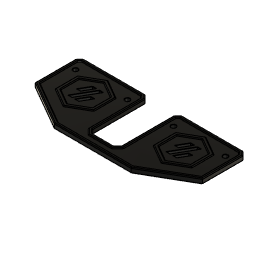
z_chain_cover (Autodesk Fusion 360 design; units mm, degrees)
Autodesk Fusion 360 part; units mm, degrees
note: some values were not read from the file. Chosen so that the rebuilt part matches the saved one: which pieces of a blend or face edit are solid. Set by a fixed rule: which sketch regions a step uses.
sketch "Sketch1" plane through (0, 0, 0) normal (0, 0, 1) x (1, 0, 0)
  line L0 (34.641, 0) -> (93.359, 0)
  line L1 (128, 20) -> (128, 51)
  line L2 (0, 51) -> (0, 20)
  line L3 (53, 51) -> (53, 11)
  line L4 (56, 8) -> (72, 8)
  line L5 (211.9099, 128.0443) -> (220.9099, 133.2405)
  line L6 (220.9099, 133.2405) -> (220.9099, 143.6328)
  line L7 (220.9099, 143.6328) -> (211.9099, 148.8289)
  line L8 (211.9099, 148.8289) -> (202.9099, 143.6328)
  line L9 (202.9099, 143.6328) -> (202.9099, 133.2405)
  line L10 (202.9099, 133.2405) -> (211.9099, 128.0443)
  line L11 (211.9099, 148.8289) -> (211.9099, 128.0443) construction
  line L12 (216.4099, 146.2309) -> (207.4099, 130.6424) construction
  line L13 (208.7265, 144.1728) -> (205.4147, 138.4366)
  line L14 (211.3245, 144.1728) -> (208.0128, 138.4366)
  line L15 (213.9226, 144.1728) -> (207.2991, 132.7005)
  line L16 (216.5207, 144.1728) -> (209.8972, 132.7005)
  line L17 (209.8972, 132.7005) -> (207.2991, 132.7005)
  line L18 (208.7265, 144.1728) -> (211.3245, 144.1728)
  line L19 (213.9226, 144.1728) -> (216.5207, 144.1728)
  line L20 (215.807, 138.4366) -> (212.4952, 132.7005)
  line L21 (212.4952, 132.7005) -> (215.0933, 132.7005)
  line L22 (215.0933, 132.7005) -> (218.4051, 138.4366)
  line L23 (215.807, 138.4366) -> (218.4051, 138.4366)
  line L24 (205.4147, 138.4366) -> (208.0128, 138.4366)
  line L25 (202.9099, 138.4366) -> (220.9099, 138.4366) construction
  line L26 (201.9099, 132.6631) -> (211.9099, 126.8896)
  line L27 (211.9099, 126.8896) -> (221.9099, 132.6631)
  line L28 (221.9099, 132.6631) -> (221.9099, 144.2101)
  line L29 (221.9099, 144.2101) -> (211.9099, 149.9836)
  line L30 (211.9099, 149.9836) -> (201.9099, 144.2101)
  line L31 (201.9099, 144.2101) -> (201.9099, 132.6631)
  line L32 (64, 46) -> (64, 0) construction
  line L33 (75, 51) -> (75, 11)
  line L34 (0, 20) -> (34.641, 0)
  line L35 (128, 20) -> (93.359, 0)
  line L36 (0, 1.75) -> (0, 22.5) construction
  line L37 (26.5, 18.2061) -> (38.5, 25.1343)
  line L38 (11.7, 40.6073) -> (11.7, 23.5177)
  line L39 (26.5, 14.9729) -> (41.3, 23.5177)
  line L40 (26.0853, 24.5943) -> (28.6834, 24.5943)
  line L41 (23.4873, 24.5943) -> (20.8892, 24.5943)
  line L42 (32.5, 42.4548) -> (20.5, 21.6702) construction
  line L43 (11.7, 23.5177) -> (26.5, 14.9729)
  line L44 (14.5, 25.1343) -> (26.5, 18.2061)
  line L45 (24.3166, 39.5307) -> (26.9147, 39.5307)
  line L46 (26.5, 49.1521) -> (11.7, 40.6073)
  line L47 (20.0048, 32.0625) -> (22.6029, 32.0625)
  line L48 (24.3166, 39.5307) -> (20.0048, 32.0625)
  line L49 (26.9147, 39.5307) -> (22.6029, 32.0625)
  line L50 (28.6834, 24.5943) -> (32.9952, 32.0625)
  line L51 (26.5, 45.9189) -> (26.5, 18.2061) construction
  line L52 (14.5, 38.9907) -> (14.5, 25.1343)
  line L53 (30.3971, 32.0625) -> (26.0853, 24.5943)
  line L54 (41.3, 23.5177) -> (41.3, 40.6073)
  line L55 (32.1108, 39.5307) -> (23.4873, 24.5943)
  line L56 (29.5127, 39.5307) -> (32.1108, 39.5307)
  line L57 (29.5127, 39.5307) -> (20.8892, 24.5943)
  line L58 (26.5, 45.9189) -> (14.5, 38.9907)
  line L59 (38.5, 38.9907) -> (26.5, 45.9189)
  line L60 (14.5, 32.0625) -> (38.5, 32.0625) construction
  line L61 (41.3, 40.6073) -> (26.5, 49.1521)
  line L62 (38.5, 25.1343) -> (38.5, 38.9907)
  line L63 (30.3971, 32.0625) -> (32.9952, 32.0625)
  line L64 (89.5, 25.1343) -> (101.5, 18.2061)
  line L65 (103.6834, 24.5943) -> (107.9952, 32.0625)
  line L66 (101.5, 45.9189) -> (89.5, 38.9907)
  line L67 (99.3166, 39.5307) -> (101.9147, 39.5307)
  line L68 (89.5, 32.0625) -> (113.5, 32.0625) construction
  line L69 (99.3166, 39.5307) -> (95.0048, 32.0625)
  line L70 (105.3971, 32.0625) -> (107.9952, 32.0625)
  line L71 (116.3, 23.5177) -> (116.3, 40.6073)
  line L72 (104.5127, 39.5307) -> (107.1108, 39.5307)
  line L73 (113.5, 38.9907) -> (101.5, 45.9189)
  line L74 (95.0048, 32.0625) -> (97.6029, 32.0625)
  line L75 (116.3, 40.6073) -> (101.5, 49.1521)
  line L76 (101.9147, 39.5307) -> (97.6029, 32.0625)
  line L77 (101.5, 49.1521) -> (86.7, 40.6073)
  line L78 (101.5, 14.9729) -> (116.3, 23.5177)
  line L79 (107.5, 42.4548) -> (95.5, 21.6702) construction
  line L80 (104.5127, 39.5307) -> (95.8892, 24.5943)
  line L81 (107.1108, 39.5307) -> (98.4873, 24.5943)
  line L82 (86.7, 40.6073) -> (86.7, 23.5177)
  line L83 (101.5, 18.2061) -> (113.5, 25.1343)
  line L84 (89.5, 38.9907) -> (89.5, 25.1343)
  line L85 (101.5, 45.9189) -> (101.5, 18.2061) construction
  line L86 (113.5, 25.1343) -> (113.5, 38.9907)
  line L87 (105.3971, 32.0625) -> (101.0853, 24.5943)
  line L88 (98.4873, 24.5943) -> (95.8892, 24.5943)
  line L89 (101.0853, 24.5943) -> (103.6834, 24.5943)
  line L90 (86.7, 23.5177) -> (101.5, 14.9729)
  circle A0 centre (6.625, 44.2) radius 1.7
  circle A1 centre (121.375, 44.2) radius 1.7
  line L91 (125, 54) -> (78, 54)
  line L92 (50, 54) -> (3, 54)
  line L93 (0, 51) -> (3, 54)
  line L94 (50, 54) -> (53, 51)
  line L95 (53, 11) -> (56, 8)
  line L96 (72, 8) -> (75, 11)
  line L97 (75, 51) -> (78, 54)
  line L98 (125, 54) -> (128, 51)
  line L99 (1.75, 0) -> (22.5, 0)
  circle A2 centre (46.375, 44.2) radius 1.7
  circle A3 centre (81.625, 44.2) radius 1.7
  line L100 (2.4, 50.0059) -> (3.9941, 51.6)
  line L101 (49.0059, 51.6) -> (3.9941, 51.6)
  line L102 (49.0059, 51.6) -> (50.6, 50.0059)
  line L103 (50.6, 50.0059) -> (50.6, 10.0059)
  line L104 (50.6, 10.0059) -> (55.0059, 5.6)
  line L105 (55.0059, 5.6) -> (72.9941, 5.6)
  line L106 (72.9941, 5.6) -> (77.4, 10.0059)
  line L107 (77.4, 50.0059) -> (77.4, 10.0059)
  line L108 (77.4, 50.0059) -> (78.9941, 51.6)
  line L109 (124.0059, 51.6) -> (78.9941, 51.6)
  line L110 (124.0059, 51.6) -> (125.6, 50.0059)
  line L111 (125.6, 21.3856) -> (125.6, 50.0059)
  line L112 (125.6, 21.3856) -> (92.7159, 2.4)
  line L113 (35.2841, 2.4) -> (92.7159, 2.4)
  line L114 (2.4, 21.3856) -> (35.2841, 2.4)
  line L115 (2.4, 50.0059) -> (2.4, 21.3856)
  point P0 (128, 54)
  point P1 (0, 54)
  point P2 (53, 54)
  point P3 (53, 8)
  point P4 (211.9099, 138.4366)
  point P5 (75, 54)
  point P6 (75, 8)
  point P7 (26.5, 32.0625)
  point P8 (101.5, 32.0625)
  point P9 (26.5, 32.0625)
  point P10 (101.5, 32.0625)
  dimension "d1" = 54
  dimension "d4" = 46
  dimension "d6" = 18
  dimension "d7" = 2.25
  dimension "d8" = 2.25
  dimension "d9" = 2.25
  dimension "d11" = 0.54
  dimension "d12" = 0.54
  dimension "d13" = 1.125
  dimension "d14" = 1
  dimension "d15" = 22
  dimension "d18" = 128
  dimension "d19" = 26.5
  dimension "d20" = 2.8
  dimension "d21" = 24
  dimension "d22" = 2.25
  dimension "d23" = 2.25
  dimension "d24" = 2.25
  dimension "d25" = 0.54
  dimension "d26" = 0.54
  dimension "d27" = 1.125
  dimension "d28" = 2.8
  dimension "d29" = 24
  dimension "d30" = 2.25
  dimension "d31" = 2.25
  dimension "d32" = 2.25
  dimension "d33" = 0.54
  dimension "d34" = 0.54
  dimension "d35" = 1.125
  dimension "d36" = 3.4
  dimension "d37" = 9.8
  dimension "d38" = 6.625
  dimension "d39" = 64
  dimension "d40" = 3
  dimension "d41" = 3
  dimension "d42" = 3
  dimension "d43" = 3
  dimension "d44" = 3
  dimension "d45" = 3
  dimension "d46" = 3
  dimension "d47" = 3
  dimension "d48" = 3
  dimension "d49" = 3
  dimension "d50" = 3
  dimension "d51" = 3
  dimension "d61" = 32.0625
  dimension "d62" = 6.625
  dimension "d63" = 20
  dimension "d64" = 30
  dimension "d65" = -2.4
  constraint horizontal L0
  constraint vertical L1
  constraint horizontal L91
  constraint vertical L2
  constraint coincident P2 L91
  constraint perpendicular L3 L91
  constraint perpendicular L3 L4
  constraint vertical L11
  constraint midpoint L7 L12.start
  constraint midpoint L10 L12.end
  constraint perpendicular L11 L18
  constraint coincident L15.start L18
  constraint horizontal L17
  constraint collinear L18 L19
  constraint parallel L12 L15
  constraint parallel L12 L16
  constraint coincident L20.start L24
  constraint parallel L16 L20
  constraint perpendicular L11 L21
  constraint parallel L20 L22
  constraint collinear L23 L24
  constraint midpoint L9 L25.start
  constraint perpendicular L6 L25
  constraint collinear L24 L25
  constraint equal L17 L21
  constraint collinear L17 L21
  constraint equal L18 L19
  constraint parallel L12 L13
  constraint midpoint L6 L25.end
  constraint symmetric P2 L32 P5
  constraint symmetric P3 L32 P6
  constraint symmetric L32 L2.end L1.start
  constraint coincident L0 L32.end
  constraint coincident origin L2
  constraint coincident origin L0
  constraint symmetric L32 L34 L35
  constraint symmetric L32 P9 P10
  constraint vertical L51
  constraint midpoint L42.start L59
  constraint midpoint L42.end L44
  constraint perpendicular L45 L51
  constraint coincident L56.start L45
  constraint horizontal L41
  constraint collinear L45 L56
  constraint parallel L42 L57
  constraint parallel L42 L55
  constraint coincident L53.start L47
  constraint parallel L53 L55
  constraint perpendicular L40 L51
  constraint parallel L50 L53
  constraint collinear L47 L63
  constraint midpoint L60.start L52
  constraint perpendicular L60 L62
  constraint collinear L47 L60
  constraint equal L40 L41
  constraint collinear L40 L41
  constraint equal L45 L56
  constraint parallel L42 L48
  constraint midpoint L60.end L62
  constraint vertical L85
  constraint midpoint L79.start L73
  constraint midpoint L79.end L64
  constraint perpendicular L67 L85
  constraint coincident L72.start L67
  constraint horizontal L88
  constraint collinear L67 L72
  constraint parallel L79 L80
  constraint parallel L79 L81
  constraint coincident L70.start L74
  constraint parallel L81 L87
  constraint perpendicular L85 L89
  constraint parallel L65 L87
  constraint collinear L70 L74
  constraint midpoint L68.start L84
  constraint perpendicular L68 L86
  constraint collinear L68 L74
  constraint equal L88 L89
  constraint collinear L88 L89
  constraint equal L67 L72
  constraint parallel L69 L79
  constraint midpoint L68.end L86
  constraint symmetric L32 A0 A1
  constraint collinear L91 L92
  constraint coincident P9 P7
  constraint coincident P10 P8
  constraint coincident P1 L2
  constraint coincident P1 L92
  constraint coincident P2 L92
  constraint coincident P3 L3
  constraint coincident P3 L4
  constraint coincident L4 P6
  constraint coincident P6 L33
  constraint coincident P5 L33
  constraint coincident P5 L91
  constraint coincident P0 L91
  constraint coincident P0 L1
  constraint equal A0 A2
  constraint horizontal A0.centre A2.centre
  constraint symmetric L32 A2 A3
  measures "d1" distance of origin P1
  measures "d4" distance of L4 L91
  measures "d6" distance of L7 L10
  measures "d7" distance of L15 L16
  measures "d8" distance of L14 L15
  measures "d9" distance of L16 L20
  measures "d11" distance of L6.end L19
  measures "d12" distance of L9.end L17
  measures "d13" distance of L12 L15
  measures "d15" distance of L3 L33
  measures "d18" distance of P0 P1
  measures "d19" distance of P9 L36
  measures "d21" distance of L44 L59
  measures "d22" distance of L55 L57
  measures "d23" distance of L49 L57
  measures "d24" distance of L53 L55
  measures "d25" distance of L59.start L56
  measures "d26" distance of L44.start L41
  measures "d27" distance of L42 L57
  measures "d29" distance of L64 L73
  measures "d30" distance of L80 L81
  measures "d31" distance of L76 L80
  measures "d32" distance of L81 L87
  measures "d33" distance of L73.start L72
  measures "d34" distance of L64.start L88
  measures "d35" distance of L79 L80
  measures "d36" diameter of A0
  measures "d37" distance of A0.centre L91
  measures "d38" distance of L2 A0.centre
  measures "d39" distance of L2 L32
  measures "d40" distance of P1 L2.start
  measures "d41" distance of P1 L92.end
  measures "d42" distance of P2 L92.start
  measures "d43" distance of P2 L3.start
  measures "d44" distance of P3 L3.end
  measures "d45" distance of P3 L4.start
  measures "d46" distance of P6 L4.end
  measures "d47" distance of P6 L33.end
  measures "d48" distance of P5 L33.start
  measures "d49" distance of P5 L91.end
  measures "d50" distance of P0 L91.start
  measures "d51" distance of P0 L1.end
  measures "d61" distance of P9 L99
  measures "d62" distance of L3 A2.centre
  measures "d63" distance of L2.end L99
  measures "d64" angle of L34 L99
extrude "Extrude1" add sketch "Sketch1" against normal blind 4 contours L0 L1 L2 L3 L4 L33 L34 L35 L91 L92 L93 L94 L95 L96 L97 L98 | L37 L44 L52 L58 L59 L62 | L38 L39 L43 L46 L54 L61 | L64 L66 L73 L83 L84 L86 | L71 L75 L77 L78 L82 L90 | L100 L101 L102 L103 L104 L105 L106 L107 L108 L109 L110 L111 L112 L113 L114 L115
extrude "Extrude2" cut sketch "Sketch1" against normal blind 0.6 contours L37 L44 L52 L58 L59 L62 | L64 L66 L73 L83 L84 L86 | A2 | A3 | L100 L101 L102 L103 L104 L105 L106 L107 L108 L109 L110 L111 L112 L113 L114 L115
chamfer "Chamfer1" distance 0.6 angle 45 4 faces at (84.1486, 26.0319, -4) (12.6333, 29.7531, 0) (92.5667, 42.9167, 0) (73.572, 0.8, 0)
chamfer "Chamfer1" distance 0.2 angle 45 32 edges at (119.79, 43.5853, -0.6) (5.04, 43.5853, -0.6) (97.1607, 35.7966, -0.6) (96.3038, 32.0625, -0.6) (99.7588, 35.7966, -0.6) (100.6156, 39.5307, -0.6) (105.8118, 39.5307, -0.6) (100.201, 32.0625, -0.6) (97.1882, 24.5943, -0.6) (102.799, 32.0625, -0.6) (102.799, 32.0625, -4) (105.8118, 39.5307, -4) (100.201, 32.0625, -4) (97.1882, 24.5943, -4) (103.2412, 28.3284, -0.6) (106.6962, 32.0625, -0.6) (105.8393, 28.3284, -0.6) (102.3844, 24.5943, -0.6) (25.6156, 39.5307, -0.6) (22.1607, 35.7966, -0.6) (21.3038, 32.0625, -0.6) (24.7588, 35.7966, -0.6) (30.8118, 39.5307, -0.6) (22.1882, 24.5943, -0.6) (25.201, 32.0625, -0.6) (27.799, 32.0625, -0.6) (28.2412, 28.3284, -0.6) (31.6962, 32.0625, -0.6) (30.8393, 28.3284, -0.6) (27.3844, 24.5943, -0.6) (44.79, 43.5853, -0.6) (80.04, 43.5853, -0.6) measured on face at (121.9164, 45.8115, -1.7333) measured on face at (5.0585, 44.8603, -1.7333) measured on face at (96.4421, 34.5519, -2.8667) measured on face at (95.8708, 32.0625, -1.7333) measured on face at (99.0401, 34.5519, -2.8667) measured on face at (100.1826, 39.5307, -1.7333) measured on face at (106.2448, 39.5307, -2.8667) measured on face at (101.6382, 34.5519, -1.7333) measured on face at (97.6212, 24.5943, -1.7333) measured on face at (104.2363, 34.5519, -2.8667) measured on face at (84.1486, 26.0319, -4) measured on face at (84.1486, 26.0319, -4) measured on face at (84.1486, 26.0319, -4) measured on face at (84.1486, 26.0319, -4) measured on face at (102.5226, 27.0837, -2.8667) measured on face at (106.2631, 32.0625, -1.7333) measured on face at (105.1207, 27.0837, -2.8667) measured on face at (101.9514, 24.5943, -1.7333) measured on face at (25.1826, 39.5307, -1.7333) measured on face at (22.8793, 37.0413, -1.7333) measured on face at (20.8708, 32.0625, -1.7333) measured on face at (25.4774, 37.0413, -1.7333) measured on face at (30.3788, 39.5307, -1.7333) measured on face at (22.6212, 24.5943, -1.7333) measured on face at (26.6382, 34.5519, -1.7333) measured on face at (29.2363, 34.5519, -1.7333) measured on face at (28.9599, 29.5731, -2.8667) measured on face at (31.2631, 32.0625, -1.7333) measured on face at (31.5579, 29.5731, -2.8667) measured on face at (26.9514, 24.5943, -1.7333) measured on face at (45.6758, 45.7496, -1.7333) measured on face at (82.1664, 45.8115, -1.7333)
equation "d7 = d6 * 0.125"
equation "d8 = d7"
equation "d9 = d7"
equation "d11 = d6 * 0.03"
equation "d12 = d11"
equation "d13 = d7 / 2"
equation "d19 = 8 / 16 * 0.5 * ( d18 - d15 )"
equation "d22 = d6 * 0.125"
equation "d23 = d7"
equation "d24 = d7"
equation "d25 = d6 * 0.03"
equation "d26 = d11"
equation "d27 = d7 / 2"
equation "d30 = d6 * 0.125"
equation "d31 = d7"
equation "d32 = d7"
equation "d33 = d6 * 0.03"
equation "d34 = d11"
equation "d35 = d7 / 2"
equation "d38 = 0.5 * 0.125 * ( d18 - d15 )"
equation "d41 = d40"
equation "d42 = d40"
equation "d43 = d42"
equation "d44 = d40"
equation "d45 = d44"
equation "d46 = d40"
equation "d47 = d46"
equation "d48 = d40"
equation "d49 = d48"
equation "d50 = d40"
equation "d51 = d50"
equation "d53 = 0 mm - 4.00 mm"
equation "d55 = 0 mm - 0.600 mm"
equation "d61 = d1 * 19 / 32"
equation "d62 = 0.5 * 0.125 * ( d18 - d15 )"
